Autodesk Fusion 360 part; units mm, degrees
(part 3 of 3)
sketch "Esquisse17" plane through (0, 0, 63) normal (0, 0, 1) x (-1, 0, 0)
  line L0 (-197, 108) -> (-186.7895, 108)
  line L1 (-186.7895, 108) -> (-186.7895, 105)
  line L2 (-186.7895, 105) -> (-176.5789, 105)
  line L3 (-176.5789, 105) -> (-176.5789, 108)
  line L4 (-176.5789, 108) -> (-166.3684, 108)
  line L5 (-166.3684, 108) -> (-166.3684, 105)
  line L6 (-166.3684, 105) -> (-156.1579, 105)
  line L7 (-156.1579, 105) -> (-156.1579, 108)
  line L8 (-156.1579, 108) -> (-145.9474, 108)
  line L9 (-145.9474, 108) -> (-145.9474, 105)
  line L10 (-145.9474, 105) -> (-135.7368, 105)
  line L11 (-135.7368, 105) -> (-135.7368, 108)
  line L12 (-135.7368, 108) -> (-125.5263, 108)
  line L13 (-125.5263, 108) -> (-125.5263, 105)
  line L14 (-125.5263, 105) -> (-115.3158, 105)
  line L15 (-115.3158, 105) -> (-115.3158, 108)
  line L16 (-115.3158, 108) -> (-105.1053, 108)
  line L17 (-105.1053, 108) -> (-105.1053, 105)
  line L18 (-105.1053, 105) -> (-94.8947, 105)
  line L19 (-94.8947, 105) -> (-94.8947, 108)
  line L20 (-94.8947, 108) -> (-84.6842, 108)
  line L21 (-84.6842, 108) -> (-84.6842, 105)
  line L22 (-84.6842, 105) -> (-74.4737, 105)
  line L23 (-74.4737, 105) -> (-74.4737, 108)
  line L24 (-74.4737, 108) -> (-64.2632, 108)
  line L25 (-64.2632, 108) -> (-64.2632, 105)
  line L26 (-64.2632, 105) -> (-54.0526, 105)
  line L27 (-54.0526, 105) -> (-54.0526, 108)
  line L28 (-54.0526, 108) -> (-43.8421, 108)
  line L29 (-43.8421, 108) -> (-43.8421, 105)
  line L30 (-43.8421, 105) -> (-33.6316, 105)
  line L31 (-33.6316, 105) -> (-33.6316, 108)
  line L32 (-33.6316, 108) -> (-23.4211, 108)
  line L33 (-23.4211, 108) -> (-23.4211, 105)
  line L34 (-23.4211, 105) -> (-13.2105, 105)
  line L35 (-13.2105, 105) -> (-13.2105, 108)
  line L36 (-13.2105, 108) -> (-3, 108)
  line L37 (-3, 108) -> (-3, 115.5263)
  line L38 (-3, 115.5263) -> (0, 115.5263)
  line L39 (0, 115.5263) -> (0, 126.0526)
  line L40 (0, 126.0526) -> (-3, 126.0526)
  line L41 (-3, 126.0526) -> (-3, 136.5789)
  line L42 (-3, 136.5789) -> (0, 136.5789)
  line L43 (0, 136.5789) -> (0, 147.1053)
  line L44 (0, 147.1053) -> (-3, 147.1053)
  line L45 (-3, 147.1053) -> (-3, 157.6316)
  line L46 (-3, 157.6316) -> (0, 157.6316)
  line L47 (0, 157.6316) -> (0, 168.1579)
  line L48 (0, 168.1579) -> (-3, 168.1579)
  line L49 (-3, 168.1579) -> (-3, 178.6842)
  line L50 (-3, 178.6842) -> (0, 178.6842)
  line L51 (0, 178.6842) -> (0, 189.2105)
  line L52 (0, 189.2105) -> (-3, 189.2105)
  line L53 (-3, 189.2105) -> (-3, 199.7368)
  line L54 (-3, 199.7368) -> (0, 199.7368)
  line L55 (0, 199.7368) -> (0, 210.2632)
  line L56 (0, 210.2632) -> (-3, 210.2632)
  line L57 (-3, 210.2632) -> (-3, 220.7895)
  line L58 (-3, 220.7895) -> (0, 220.7895)
  line L59 (0, 220.7895) -> (0, 231.3158)
  line L60 (0, 231.3158) -> (-3, 231.3158)
  line L61 (-3, 231.3158) -> (-3, 241.8421)
  line L62 (-3, 241.8421) -> (0, 241.8421)
  line L63 (0, 241.8421) -> (0, 252.3684)
  line L64 (0, 252.3684) -> (-3, 252.3684)
  line L65 (-3, 252.3684) -> (-3, 262.8947)
  line L66 (-3, 262.8947) -> (0, 262.8947)
  line L67 (0, 262.8947) -> (0, 273.4211)
  line L68 (0, 273.4211) -> (-3, 273.4211)
  line L69 (-3, 273.4211) -> (-3, 283.9474)
  line L70 (-3, 283.9474) -> (0, 283.9474)
  line L71 (0, 283.9474) -> (0, 294.4737)
  line L72 (0, 294.4737) -> (-3, 294.4737)
  line L73 (-3, 294.4737) -> (-3, 302)
  line L74 (-3, 302) -> (-13.2105, 302)
  line L75 (-13.2105, 302) -> (-13.2105, 305)
  line L76 (-13.2105, 305) -> (-23.4211, 305)
  line L77 (-23.4211, 305) -> (-23.4211, 302)
  line L78 (-23.4211, 302) -> (-33.6316, 302)
  line L79 (-33.6316, 302) -> (-33.6316, 305)
  line L80 (-33.6316, 305) -> (-43.8421, 305)
  line L81 (-43.8421, 305) -> (-43.8421, 302)
  line L82 (-43.8421, 302) -> (-54.0526, 302)
  line L83 (-54.0526, 302) -> (-54.0526, 305)
  line L84 (-54.0526, 305) -> (-64.2632, 305)
  line L85 (-64.2632, 305) -> (-64.2632, 302)
  line L86 (-64.2632, 302) -> (-74.4737, 302)
  line L87 (-74.4737, 302) -> (-74.4737, 305)
  line L88 (-74.4737, 305) -> (-84.6842, 305)
  line L89 (-84.6842, 305) -> (-84.6842, 302)
  line L90 (-84.6842, 302) -> (-94.8947, 302)
  line L91 (-94.8947, 302) -> (-94.8947, 305)
  line L92 (-94.8947, 305) -> (-105.1053, 305)
  line L93 (-105.1053, 305) -> (-105.1053, 302)
  line L94 (-105.1053, 302) -> (-115.3158, 302)
  line L95 (-115.3158, 302) -> (-115.3158, 305)
  line L96 (-115.3158, 305) -> (-125.5263, 305)
  line L97 (-125.5263, 305) -> (-125.5263, 302)
  line L98 (-125.5263, 302) -> (-135.7368, 302)
  line L99 (-135.7368, 302) -> (-135.7368, 305)
  line L100 (-135.7368, 305) -> (-145.9474, 305)
  line L101 (-145.9474, 305) -> (-145.9474, 302)
  line L102 (-145.9474, 302) -> (-156.1579, 302)
  line L103 (-156.1579, 302) -> (-156.1579, 305)
  line L104 (-156.1579, 305) -> (-166.3684, 305)
  line L105 (-166.3684, 305) -> (-166.3684, 302)
  line L106 (-166.3684, 302) -> (-176.5789, 302)
  line L107 (-176.5789, 302) -> (-176.5789, 305)
  line L108 (-176.5789, 305) -> (-186.7895, 305)
  line L109 (-186.7895, 305) -> (-186.7895, 302)
  line L110 (-186.7895, 302) -> (-197, 302)
  line L111 (-197, 302) -> (-197, 294.4737)
  line L112 (-197, 294.4737) -> (-200, 294.4737)
  line L113 (-200, 294.4737) -> (-200, 283.9474)
  line L114 (-200, 283.9474) -> (-197, 283.9474)
  line L115 (-197, 283.9474) -> (-197, 273.4211)
  line L116 (-197, 273.4211) -> (-200, 273.4211)
  line L117 (-200, 273.4211) -> (-200, 262.8947)
  line L118 (-200, 262.8947) -> (-197, 262.8947)
  line L119 (-197, 262.8947) -> (-197, 252.3684)
  line L120 (-197, 252.3684) -> (-200, 252.3684)
  line L121 (-200, 252.3684) -> (-200, 241.8421)
  line L122 (-200, 241.8421) -> (-197, 241.8421)
  line L123 (-197, 241.8421) -> (-197, 231.3158)
  line L124 (-197, 231.3158) -> (-200, 231.3158)
  line L125 (-200, 231.3158) -> (-200, 220.7895)
  line L126 (-200, 220.7895) -> (-197, 220.7895)
  line L127 (-197, 220.7895) -> (-197, 210.2632)
  line L128 (-197, 210.2632) -> (-200, 210.2632)
  line L129 (-200, 210.2632) -> (-200, 199.7368)
  line L130 (-200, 199.7368) -> (-197, 199.7368)
  line L131 (-197, 199.7368) -> (-197, 189.2105)
  line L132 (-197, 189.2105) -> (-200, 189.2105)
  line L133 (-200, 189.2105) -> (-200, 178.6842)
  line L134 (-200, 178.6842) -> (-197, 178.6842)
  line L135 (-197, 178.6842) -> (-197, 168.1579)
  line L136 (-197, 168.1579) -> (-200, 168.1579)
  line L137 (-200, 168.1579) -> (-200, 157.6316)
  line L138 (-200, 157.6316) -> (-197, 157.6316)
  line L139 (-197, 157.6316) -> (-197, 147.1053)
  line L140 (-197, 147.1053) -> (-200, 147.1053)
  line L141 (-200, 147.1053) -> (-200, 136.5789)
  line L142 (-200, 136.5789) -> (-197, 136.5789)
  line L143 (-197, 136.5789) -> (-197, 126.0526)
  line L144 (-197, 126.0526) -> (-200, 126.0526)
  line L145 (-200, 126.0526) -> (-200, 115.5263)
  line L146 (-200, 115.5263) -> (-197, 115.5263)
  line L147 (-197, 115.5263) -> (-197, 108)
sketch "Esquisse18" plane through (0, 0, 3) normal (0, 0, -1) x (1, 0, 0)
  circle A0 centre (175, 130) radius 10
  circle A1 centre (175, 280) radius 10
  circle A2 centre (25, 130) radius 10
  circle A3 centre (25, 280) radius 10
  line L0 (21.0526, 305) -> (10.5263, 305)
  line L1 (10.5263, 305) -> (10.5263, 302)
  line L2 (10.5263, 302) -> (3, 302)
  line L3 (3, 302) -> (3, 294.4737)
  line L4 (3, 294.4737) -> (0, 294.4737)
  line L5 (0, 294.4737) -> (0, 283.9474)
  line L6 (0, 283.9474) -> (3, 283.9474)
  line L7 (3, 283.9474) -> (3, 273.4211)
  line L8 (3, 273.4211) -> (0, 273.4211)
  line L9 (0, 273.4211) -> (0, 262.8947)
  line L10 (0, 262.8947) -> (3, 262.8947)
  line L11 (3, 262.8947) -> (3, 252.3684)
  line L12 (3, 252.3684) -> (0, 252.3684)
  line L13 (0, 252.3684) -> (0, 241.8421)
  line L14 (0, 241.8421) -> (3, 241.8421)
  line L15 (3, 241.8421) -> (3, 231.3158)
  line L16 (3, 231.3158) -> (0, 231.3158)
  line L17 (0, 231.3158) -> (0, 220.7895)
  line L18 (0, 220.7895) -> (3, 220.7895)
  line L19 (3, 220.7895) -> (3, 210.2632)
  line L20 (3, 210.2632) -> (0, 210.2632)
  line L21 (0, 210.2632) -> (0, 199.7368)
  line L22 (0, 199.7368) -> (3, 199.7368)
  line L23 (3, 199.7368) -> (3, 189.2105)
  line L24 (3, 189.2105) -> (0, 189.2105)
  line L25 (0, 189.2105) -> (0, 178.6842)
  line L26 (0, 178.6842) -> (3, 178.6842)
  line L27 (3, 178.6842) -> (3, 168.1579)
  line L28 (3, 168.1579) -> (0, 168.1579)
  line L29 (0, 168.1579) -> (0, 157.6316)
  line L30 (0, 157.6316) -> (3, 157.6316)
  line L31 (3, 157.6316) -> (3, 147.1053)
  line L32 (3, 147.1053) -> (0, 147.1053)
  line L33 (0, 147.1053) -> (0, 136.5789)
  line L34 (0, 136.5789) -> (3, 136.5789)
  line L35 (3, 136.5789) -> (3, 126.0526)
  line L36 (3, 126.0526) -> (0, 126.0526)
  line L37 (0, 126.0526) -> (0, 115.5263)
  line L38 (0, 115.5263) -> (3, 115.5263)
  line L39 (3, 115.5263) -> (3, 108)
  line L40 (3, 108) -> (10.5263, 108)
  line L41 (10.5263, 108) -> (10.5263, 105)
  line L42 (10.5263, 105) -> (21.0526, 105)
  line L43 (21.0526, 105) -> (21.0526, 108)
  line L44 (21.0526, 108) -> (31.5789, 108)
  line L45 (31.5789, 108) -> (31.5789, 105)
  line L46 (31.5789, 105) -> (42.1053, 105)
  line L47 (42.1053, 105) -> (42.1053, 108)
  line L48 (42.1053, 108) -> (52.6316, 108)
  line L49 (52.6316, 108) -> (52.6316, 105)
  line L50 (52.6316, 105) -> (63.1579, 105)
  line L51 (63.1579, 105) -> (63.1579, 108)
  line L52 (63.1579, 108) -> (73.6842, 108)
  line L53 (73.6842, 108) -> (73.6842, 105)
  line L54 (73.6842, 105) -> (84.2105, 105)
  line L55 (84.2105, 105) -> (84.2105, 108)
  line L56 (84.2105, 108) -> (94.7368, 108)
  line L57 (94.7368, 108) -> (94.7368, 105)
  line L58 (94.7368, 105) -> (105.2632, 105)
  line L59 (105.2632, 105) -> (105.2632, 108)
  line L60 (105.2632, 108) -> (115.7895, 108)
  line L61 (115.7895, 108) -> (115.7895, 105)
  line L62 (115.7895, 105) -> (126.3158, 105)
  line L63 (126.3158, 105) -> (126.3158, 108)
  line L64 (126.3158, 108) -> (136.8421, 108)
  line L65 (136.8421, 108) -> (136.8421, 105)
  line L66 (136.8421, 105) -> (147.3684, 105)
  line L67 (147.3684, 105) -> (147.3684, 108)
  line L68 (147.3684, 108) -> (157.8947, 108)
  line L69 (157.8947, 108) -> (157.8947, 105)
  line L70 (157.8947, 105) -> (168.4211, 105)
  line L71 (168.4211, 105) -> (168.4211, 108)
  line L72 (168.4211, 108) -> (178.9474, 108)
  line L73 (178.9474, 108) -> (178.9474, 105)
  line L74 (178.9474, 105) -> (189.4737, 105)
  line L75 (189.4737, 105) -> (189.4737, 108)
  line L76 (189.4737, 108) -> (197, 108)
  line L77 (197, 108) -> (197, 115.5263)
  line L78 (197, 115.5263) -> (200, 115.5263)
  line L79 (200, 115.5263) -> (200, 126.0526)
  line L80 (200, 126.0526) -> (197, 126.0526)
  line L81 (197, 126.0526) -> (197, 136.5789)
  line L82 (197, 136.5789) -> (200, 136.5789)
  line L83 (200, 136.5789) -> (200, 147.1053)
  line L84 (200, 147.1053) -> (197, 147.1053)
  line L85 (197, 147.1053) -> (197, 157.6316)
  line L86 (197, 157.6316) -> (200, 157.6316)
  line L87 (200, 157.6316) -> (200, 168.1579)
  line L88 (200, 168.1579) -> (197, 168.1579)
  line L89 (197, 168.1579) -> (197, 178.6842)
  line L90 (197, 178.6842) -> (200, 178.6842)
  line L91 (200, 178.6842) -> (200, 189.2105)
  line L92 (200, 189.2105) -> (197, 189.2105)
  line L93 (197, 189.2105) -> (197, 199.7368)
  line L94 (197, 199.7368) -> (200, 199.7368)
  line L95 (200, 199.7368) -> (200, 210.2632)
  line L96 (200, 210.2632) -> (197, 210.2632)
  line L97 (197, 210.2632) -> (197, 220.7895)
  line L98 (197, 220.7895) -> (200, 220.7895)
  line L99 (200, 220.7895) -> (200, 231.3158)
  line L100 (200, 231.3158) -> (197, 231.3158)
  line L101 (197, 231.3158) -> (197, 241.8421)
  line L102 (197, 241.8421) -> (200, 241.8421)
  line L103 (200, 241.8421) -> (200, 252.3684)
  line L104 (200, 252.3684) -> (197, 252.3684)
  line L105 (197, 252.3684) -> (197, 262.8947)
  line L106 (197, 262.8947) -> (200, 262.8947)
  line L107 (200, 262.8947) -> (200, 273.4211)
  line L108 (200, 273.4211) -> (197, 273.4211)
  line L109 (197, 273.4211) -> (197, 283.9474)
  line L110 (197, 283.9474) -> (200, 283.9474)
  line L111 (200, 283.9474) -> (200, 294.4737)
  line L112 (200, 294.4737) -> (197, 294.4737)
  line L113 (197, 294.4737) -> (197, 302)
  line L114 (197, 302) -> (189.4737, 302)
  line L115 (189.4737, 302) -> (189.4737, 305)
  line L116 (189.4737, 305) -> (178.9474, 305)
  line L117 (178.9474, 305) -> (178.9474, 302)
  line L118 (178.9474, 302) -> (168.4211, 302)
  line L119 (168.4211, 302) -> (168.4211, 305)
  line L120 (168.4211, 305) -> (157.8947, 305)
  line L121 (157.8947, 305) -> (157.8947, 302)
  line L122 (157.8947, 302) -> (147.3684, 302)
  line L123 (147.3684, 302) -> (147.3684, 305)
  line L124 (147.3684, 305) -> (136.8421, 305)
  line L125 (136.8421, 305) -> (136.8421, 302)
  line L126 (136.8421, 302) -> (126.3158, 302)
  line L127 (126.3158, 302) -> (126.3158, 305)
  line L128 (126.3158, 305) -> (115.7895, 305)
  line L129 (115.7895, 305) -> (115.7895, 302)
  line L130 (115.7895, 302) -> (105.2632, 302)
  line L131 (105.2632, 302) -> (105.2632, 305)
  line L132 (105.2632, 305) -> (94.7368, 305)
  line L133 (94.7368, 305) -> (94.7368, 302)
  line L134 (94.7368, 302) -> (84.2105, 302)
  line L135 (84.2105, 302) -> (84.2105, 305)
  line L136 (84.2105, 305) -> (73.6842, 305)
  line L137 (73.6842, 305) -> (73.6842, 302)
  line L138 (73.6842, 302) -> (63.1579, 302)
  line L139 (63.1579, 302) -> (63.1579, 305)
  line L140 (63.1579, 305) -> (52.6316, 305)
  line L141 (52.6316, 305) -> (52.6316, 302)
  line L142 (52.6316, 302) -> (42.1053, 302)
  line L143 (42.1053, 302) -> (42.1053, 305)
  line L144 (42.1053, 305) -> (31.5789, 305)
  line L145 (31.5789, 305) -> (31.5789, 302)
  line L146 (31.5789, 302) -> (21.0526, 302)
  line L147 (21.0526, 302) -> (21.0526, 305)
  circle A4 centre (100, 205) radius 10
extrude "Extrusion16" cut sketch "Esquisse18" against normal blind 3 contours A4 bodies 6
equation "epaisseur = 3 mm"
equation "largeur = 200 mm"
equation "longueur = 200 mm"
equation "hauteur1 = 130 mm"
equation "d9 = longueur"
equation "d10 = largeur"
equation "d11 = longueur / 19"
equation "d12 = epaisseur"
equation "d15 = longueur / 19"
equation "d16 = longueur - epaisseur"
equation "d17 = epaisseur"
equation "d18 = longueur / 19"
equation "d21 = longueur - epaisseur"
equation "d22 = longueur / 19"
equation "d23 = epaisseur"
equation "d26 = largeur"
equation "d27 = hauteur1"
equation "d28 = -epaisseur"
equation "d30 = epaisseur"
equation "d31 = hauteur1 / 9"
equation "d34 = longueur - epaisseur"
equation "d35 = hauteur1 / 9"
equation "d36 = -epaisseur"
equation "d41 = longueur"
equation "d42 = hauteur1"
equation "d43 = -epaisseur"
equation "hauteur2 = 60 mm"
equation "d48 = largeur"
equation "d49 = longueur"
equation "d50 = largeur / 19"
equation "d51 = epaisseur"
equation "d54 = largeur / 19"
equation "d55 = largeur - epaisseur"
equation "d56 = epaisseur"
equation "d57 = largeur / 19"
equation "d60 = longueur - epaisseur"
equation "d61 = largeur / 19"
equation "d62 = epaisseur"
equation "d65 = largeur"
equation "d66 = hauteur2"
equation "d67 = -epaisseur"
equation "d69 = epaisseur"
equation "d70 = hauteur2 / 5"
equation "d73 = largeur - epaisseur"
equation "d74 = hauteur2 / 5"
equation "d75 = -epaisseur"
equation "d77 = largeur / 19"
equation "d78 = epaisseur"
equation "d81 = largeur / 19"
equation "d83 = -epaisseur"
equation "d88 = largeur"
equation "d89 = hauteur2"
equation "d90 = -epaisseur"
equation "d92 = ( largeur - 2 * epaisseur ) / 19"
equation "d93 = epaisseur"
equation "d96 = ( largeur - 2 * epaisseur ) / 19"
equation "d98 = -epaisseur"
equation "d103 = longueur"
equation "d104 = longueur"
equation "d105 = -epaisseur"
equation "d119 = -epaisseur"
equation "d126 = -epaisseur"
equation "d133 = -epaisseur"
equation "d140 = -epaisseur"
equation "d147 = -epaisseur"
